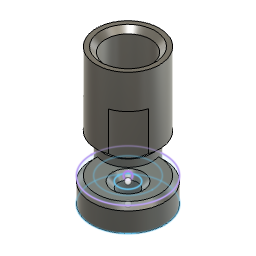
wall mount elastic lamp (Autodesk Fusion 360 design; units mm, degrees)
Autodesk Fusion 360 part; units mm, degrees
note: some values were not read from the file. Set by a fixed rule: which face or edge a step refers to.
sketch "Sketch1" plane through (0, 0, 0) normal (0, 1, 0) x (1, 0, 0)
  circle A0 centre (-170, -40) radius 5
  circle A1 centre (-165, -45) radius 7.5
  dimension "d248" = 10
  dimension "d249" = 15
  measures "d248" diameter of A0
  measures "d249" diameter of A1
extrude "Extrude2" add sketch "Sketch1" along normal blind 16 contours A0 A1 | A0 A1 picked at (-169.3882, -41.3612) picked at (-170.8309, -38.1611) makes body 1
extrude "Extrude1" add sketch "Sketch1" along normal blind 5 separate body contours A0 A1 | A0 A1 picked at (-169.3882, -41.3612) picked at (-161.994, -48.0662) makes body 2
sketch "Sketch2" plane through (0, 16, 0) normal (0, 1, 0) x (-1, 0, 0)
  circle A0 centre (170, 40) radius 5
  circle A1 centre (170, 40) radius 1.9
  dimension "d254" = 3.8
  constraint concentric A0 A1
  measures "d254" diameter of A1
sketch "Sketch3" plane through (0, 5, 0) normal (0, 1, 0) x (-1, 0, 0)
  circle A0 centre (165, 45) radius 7.5
  circle A1 centre (164, 46) radius 2
  circle A2 centre (165, 45) radius 7.5
  dimension "d257" = 4
  dimension "d263" = 15
  measures "d257" diameter of A1
  measures "d263" diameter of A2
hole "Hole1" at (-164, 5, 46) direction (0, -1, 0) diameter 4 depth 6 tip angle 118 countersink diameter 6.4 countersink angle 90 bodies 2
chamfer "Chamfer1" distance 1 angle 45 1 edges at (-171.9925, 5, 47.7121) on bodies 1 2
chamfer "Chamfer1" distance 1 angle 45 1 edges at (-174.6616, 16, 41.8081) on bodies 1 2
ref_plane "WorkPlane1" through (-170, 23, 40) normal (0, 1, 0) x (1, 0, 0)
sketch "Sketch5" plane through (-170, 23, 40) normal (0, 1, 0) x (1, 0, 0)
  circle A0 centre (0, 0) radius 6.5
  dimension "d272" = 13
  constraint coincident A0.centre origin
  measures "d272" diameter of A0
extrude "Extrude4" add sketch "Sketch5" against normal blind 15 bodies 1
shell "Shell1" thickness 1.9 removed faces 1 at (-168.0479, 23, 40.9401) on bodies 1
chamfer "Chamfer2" distance 1 angle 45 1 edges at (-174.2887, 23, 38.3366) on bodies 1
extrude "Extrude5" add 1 faces at (-169.7701, 1.9, 41.0074) along direction (0, 1, 0) blind 9 on bodies 1 bodies 1 2
sketch "Sketch6" plane through (0, 5, 0) normal (0, 1, 0) x (-1, 0, 0)
  circle A0 centre (165, 45) radius 1.7495
  ellipse E0 centre (165, 45) end of major axis (166.268, 43.7947) minor radius 4.1608
  line L0 (163.732, 46.2053) -> (166.268, 43.7947)
  line L1 (162.1334, 41.9842) -> (167.8666, 48.0158)
  constraint concentric A0 E0
  constraint coincident E0 L0.start
  constraint coincident E0 L0.end
  constraint coincident E0 L1.start
  constraint coincident E0 L1.end
extrude "Extrude6" cut sketch "Sketch6" along normal blind 11 bodies 1
chamfer "Chamfer3" distance 1.5 angle 45 1 edges at (-174.6616, 8, 38.1919) on bodies 1
extrude "Extrude7" cut 1 faces at (-169.7701, 10.9, 41.0074) along direction (0, -1, 0) blind 1 on bodies 1 bodies 1
